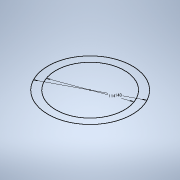
# Autodesk Inventor part: TurnTable_140_Outer
Saved by Autodesk Inventor 2022 (Build 260153000, 153)
## iProperties
Created: 2021-11-29
Part Number: TurnTable_140_Outer
Material: 鋼、合金
Document SubType Name: Modeling
Designer: satot
Density: 7.73 g/cm^3
Appearance: 半つや出し
Author: satot
Autodesk Inventor part; units mm, degrees
ref_plane "YZ Plane" through (0, 0, 0) normal (1, 0, 0) x (0, 1, 0)
ref_plane "XZ Plane" through (0, 0, 0) normal (0, 1, 0) x (-1, 0, 0)
ref_plane "XY Plane" through (0, 0, 0) normal (0, 0, 1) x (1, 0, 0)
sketch "スケッチ1" plane through (0, 0, 0) normal (0, 0, 1) x (1, 0, 0)
  circle A0 centre (0, 0) radius 70
  circle A1 centre (0, 0) radius 57
  dimension "d0" = 140
  dimension "d1" = 114
  constraints: 2 centre point, 2 coincident
  measures "d0" diameter of A0
  measures "d1" diameter of A1
extrude "押し出し1" add sketch "スケッチ1" along normal blind 8.2
sketch "スケッチ2" plane through (0, 0, 8.2) normal (0, 0, 1) x (1, 0, 0)
  point P0 (0, 0)
  point P1 (-64, 0)
  point P2 (0, -64)
  point P3 (64, 0)
  point P4 (0, 64)
  dimension "d4" = 64
  dimension "d7" = 360
  constraints: 1 horizontal alignment, 5 other
  measures "d4" distance of point (0, 0) point (-64, 0)
hole "穴1" at (-64, 0, 8.2) at (0, -64, 8.2) at (64, 0, 8.2) at (0, 64, 8.2) direction (0, 0, -1) diameter 4.4 end through all countersink diameter 10 countersink angle 90
fillet "フィレット1" radius 0.5 4 edges at (-70, 0, 0) (-57, 0, 0) (-70, 0, 8.2) (-57, 0, 8.2)
